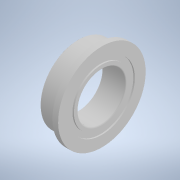
# Autodesk Inventor part: C-FL675ZZ
Saved by Autodesk Inventor 2021 (Build 250183000, 183)
## iProperties
Created: 2025-06-07
Part Number: C-FL675ZZ
Material: Generic
Catalog Web Link: www.cadenas.de
Description: C-FL673ZZ, C-FL683ZZ, C-FL693ZZ, C-FL603ZZ, C-FL623ZZ, C-FL674ZZ, C-FL684ZZ, C-FL694ZZ, C-FL604ZZ, C-FL624ZZ, C-FL675ZZ, C-FL685ZZ, C-FL695ZZ, C-FL605ZZ, C-FL625ZZ, C-FL676ZZ, C-FL686ZZ, C-FL696ZZ, C-FL606ZZ, C-FL626ZZ, C-FL678ZZ, C-FL688ZZ, C-FL698ZZ, C-FL608ZZ-C-VALUE Medium Accuracy Small Deep Groove Ball Bearings with Flange - Double Shielded - C-FL673ZZ
Vendor: MISUMI
Document SubType Name: Modeling
Designer: psAdmin
Manufacturer: MISUMI
Mass: 0.0830445 g
Surface Area: 2.07687 cm^2
Volume: 0.0830445 cm^3
Density: 1 g/cm^3
Appearance: PSOLRGB-175-175-175
Category: PARTsolutions
Company: MISUMI
Title: C-FL675ZZ
Author: Cadenas PARTsolutions
Comments: C-VALUE Medium Accuracy Small Deep Groove Ball Bearings with Flange - Double Shielded - C-FL673ZZ
PSOL_IDENT_0: {$CADENAS_DATA/23d-libs/misumi/metric/12_bearing_holders/c_fl673zz.prj},415 {VTYP=3D},{NB=C-FL675ZZ}
PSOL_IDENT_1: ,{LINA=C-FL675ZZ},{NN=C-FL673ZZ, C-FL683ZZ, C-FL693ZZ, C-FL603ZZ, C-FL623ZZ, C-FL674ZZ, C-FL684ZZ, C
PSOL_IDENT_2: -FL694ZZ, C-FL604ZZ, C-FL624ZZ, C-FL675ZZ, C-FL685ZZ, C-FL695ZZ, C-FL605ZZ, C-FL625ZZ, C-FL676ZZ, C-
PSOL_IDENT_3: FL686ZZ, C-FL696ZZ, C-FL606ZZ, C-FL626ZZ, C-FL678ZZ, C-FL688ZZ, C-FL698ZZ, C-FL608ZZ},{DATE=29.05.20
PSOL_IDENT_4: 23 02:13:13},{GEOMDATE=28.10.2019 01:37:04},{VERSION=},{LINEID=810},{WBVAR=},{WBNUMERIC=}  {NB=C-FL6
PSOL_IDENT_5: 75ZZ},{LINA=C-FL675ZZ},{KT=DUMMY},{PN=C-FL675ZZ},{TS=C-FL675ZZ},{DD=5},{D=8},{B=2.5},{D1=9.2},{C=0.6
PSOL_IDENT_6: },{RR=0.10},{DD1=5.88},{B1=0.15},{D2=6.92}
NB: C-FL675ZZ
NN: C-FL673ZZ, C-FL683ZZ, C-FL693ZZ, C-FL603ZZ, C-FL623ZZ, C-FL674ZZ, C-FL684ZZ, C-FL694ZZ, C-FL604ZZ, C-FL624ZZ, C-FL675ZZ, C-FL685ZZ, C-FL695ZZ, C-FL605ZZ, C-FL625ZZ, C-FL676ZZ, C-FL686ZZ, C-FL696ZZ, C-FL606ZZ, C-FL626ZZ, C-FL678ZZ, C-FL688ZZ, C-FL698ZZ, C-FL608ZZ
NT: C-VALUE Medium Accuracy Small Deep Groove Ball Bearings with Flange - Double Shielded - C-FL673ZZ
NBSYN: $PN.
LINA: C-FL675ZZ
CATALOG: Misumi
PN: C-FL675ZZ
TS: C-FL675ZZ
DD: 5
D: 8
B: 2.5
D1: 9.2
C: 0.6
RR: 0.1
SUPPLIER: MISUMI
ARTICLENO: C-FL675ZZ
BOMINFO: C-FL675ZZ
CREATOR: CADENAS GmbH
Autodesk Inventor part; units mm, degrees
ref_plane "YZ Plane" through (0, 0, 0) normal (1, 0, 0) x (0, 1, 0)
ref_plane "XZ Plane" through (0, 0, 0) normal (0, 1, 0) x (-1, 0, 0)
ref_plane "XY Plane" through (0, 0, 0) normal (0, 0, 1) x (1, 0, 0)
sketch "_____1" plane through (0, 0, 0) normal (0, 0, 1) x (1, 0, 0)
  line L0 (50, 0) -> (-50, 0)
  line L1 (-1.25, 0) -> (-1.25, 2.94)
  line L2 (-1.25, 2.94) -> (-1.1, 2.94)
  line L3 (-1.1, 2.94) -> (-1.1, 3.46)
  line L4 (-1.1, 3.46) -> (-1.25, 3.46)
  line L5 (-1.25, 3.46) -> (-1.25, 3.9)
  arc A0 (-1.15, 4) -> (-1.25, 3.9) centre (-1.15, 3.9) ccw
  line L6 (-1.15, 4) -> (0.65, 4)
  line L7 (0.65, 4) -> (0.65, 4.6)
  line L8 (0.65, 4.6) -> (1.25, 4.6)
  line L9 (1.25, 4.6) -> (1.25, 3.46)
  line L10 (1.25, 3.46) -> (1.1, 3.46)
  line L11 (1.1, 3.46) -> (1.1, 2.94)
  line L12 (1.1, 2.94) -> (1.25, 2.94)
  line L13 (1.25, 2.94) -> (1.25, 0)
  line L14 (1.25, 0) -> (-1.25, 0)
  constraints: 30 end point, 2 point on circle, 1 centre point
revolve "Revolution1" add sketch "_____1" angle 360 about axis through (50, 0, 0) along (1, 0, 0)
sketch "_____2" plane through (0, 0, 0) normal (0, 0, 1) x (1, 0, 0)
  line L0 (50, 0) -> (-50, 0)
  line L1 (-1.25, 0) -> (-1.25, 2.6)
  arc A0 (-1.25, 2.6) -> (-1.15, 2.5) centre (-1.15, 2.6) ccw
  line L2 (-1.15, 2.5) -> (1.15, 2.5)
  arc A1 (1.15, 2.5) -> (1.25, 2.6) centre (1.15, 2.6) ccw
  line L3 (1.25, 2.6) -> (1.25, 0)
  line L4 (1.25, 0) -> (-1.25, 0)
  constraints: 10 end point, 4 point on circle, 2 centre point
revolve "Revolution2" cut sketch "_____2" angle 360 about axis through (50, 0, 0) along (1, 0, 0)
body "Solid1"
